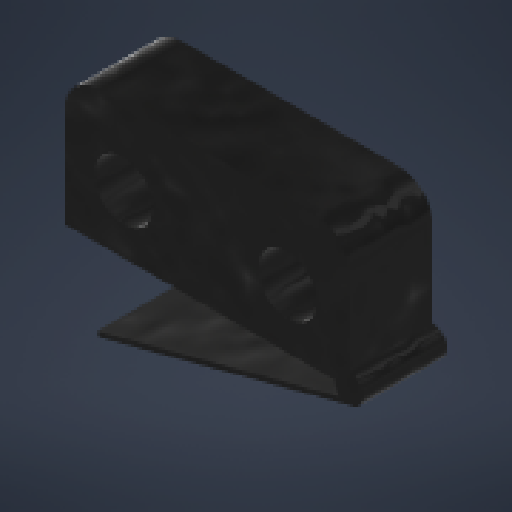
# Autodesk Inventor part: công tắc hành trình
Saved by Autodesk Inventor 2027.1 (Build 311270010, 270A)
## iProperties
Created: 2026-08-19
Part Number: công tắc hành trình
Material: Generic
Document SubType Name: Sheet Metal
Designer: MSI
Density: 1 g/cm^3
Sheet Metal Rule: Default_mm
Appearance: Fine Textured - Black
Author: MSI
Autodesk Inventor part; units mm, degrees
ref_plane "YZ Plane" through (0, 0, 0) normal (1, 0, 0) x (0, 1, 0)
ref_plane "XZ Plane" through (0, 0, 0) normal (0, 1, 0) x (-1, 0, 0)
ref_plane "XY Plane" through (0, 0, 0) normal (0, 0, 1) x (1, 0, 0)
sketch "Sketch1" plane through (0, 0, 0) normal (0, 0, 1) x (1, 0, 0)
  line L0 (0, 0) -> (17, 0)
  line L1 (17, 0.8671) -> (17, 6)
  line L2 (15, 8) -> (2, 8)
  line L3 (0, 6) -> (0, 0)
  line L4 (17, -0.8671) -> (2, -4.8546)
  line L5 (2, -4.8546) -> (1.9259, -4.5758)
  line L6 (1.9259, -4.5758) -> (16.4929, -0.7033)
  arc A0 (17, -0.8671) -> (17, 0.8671) centre (17, 0) ccw
  arc A1 (16.1329, 0) -> (16.4929, -0.7033) centre (17, 0) ccw
  arc A2 (2, 8) -> (0, 6) centre (2, 6) ccw
  arc A3 (17, 6) -> (15, 8) centre (15, 6) ccw
  point P0 (17, 8)
  point P1 (0, 8)
  dimension "d0" = 17
  dimension "d1" = 8
  dimension "d9" = 2
  constraints: 14 end point, 8 point on circle, 5 point on line, 4 centre point, 4 tangent, 3 perpendicular, 2 parallel, 1 coincident, 1 equal radius, 1 horizontal
  measures "d0" distance of point (0, 8) point (17, 8)
  measures "d1" distance of L0.end point (17, 8)
  measures "d9" radius of A2
extrude "Extrusion1" add sketch "Sketch1" along normal blind 5
sketch "Sketch2" plane through (0, 0, 5) normal (0, 0, 1) x (1, 0, 0)
  circle A0 centre (3.5, 3.5) radius 1.75
  circle A1 centre (13.3, 3.5) radius 1.75
  line L0 (0, 0) -> (16.1329, 0) projected
  line L1 (0, 6) -> (0, 0) projected
  dimension "d4" = 3.5
  dimension "d5" = 3.5
  dimension "d6" = 9.8
  dimension "d10" = 3.5
  dimension "d11" = 3.5
  dimension "d12" = 3.5
  constraints: 2 centre point
  measures "d4" diameter of A0
  measures "d5" diameter of A1
  measures "d6" distance of A1.centre A0.centre
  measures "d10" distance from line of L0 A0.centre
  measures "d11" distance from line of L0 A1.centre
  measures "d12" distance from line of L1 A0.centre
extrude "Extrusion2" cut sketch "Sketch2" against normal blind 5
equation "\"BendRadius\" = Thickness"
equation "\"BendReliefWidth\" = Thickness"
equation "\"BendReliefDepth\" = 0.5 * Thickness"
equation "\"CornerReliefSize\" = 4 * Thickness"
equation "\"MinimumRemnant\" = 2 * Thickness"
equation "\"TransitionRadius\" = BendRadius"
equation "\"JacobiRadiusSize\" = BendRadius"
equation "\"GapSize\" = Thickness"
equation "\"Thickness\" = 0.5"
body "Solid1"
